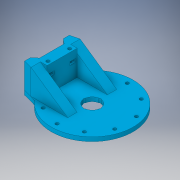
# Autodesk Inventor part: 000.302 - Кожух
Saved by Autodesk Inventor 2019 (Build 230136000, 136)
## iProperties
Created: 2020-03-19
Part Number: 000.302 - Кожух
Material: Пластик АБС
Document SubType Name: Modeling
Designer: user
Density: 1.06 g/cm^3
Appearance: Небесно-голубой — нейтральный
Author: user
Autodesk Inventor part; units mm, degrees
ref_plane "YZ Plane" through (0, 0, 0) normal (1, 0, 0) x (0, 1, 0)
ref_plane "XZ Plane" through (0, 0, 0) normal (0, 1, 0) x (-1, 0, 0)
sketch "Эскиз12" plane through (0, 0, 0) normal (0, 1, 0) x (-1, 0, 0)
  line L0 (114.5, 15) -> (114.5, 11.5)
  line L1 (114.5, 11.5) -> (114.5, -11.5)
  line L2 (114.5, -11.5) -> (114.5, -15)
  line L3 (114.5, -15) -> (108.5, -20.1)
  line L4 (108.5, -20.1) -> (55.4, -20.1)
  line L5 (55.4, -20.1) -> (49.4, -15)
  line L6 (49.4, -15) -> (49.4, 15)
  line L7 (49.4, 15) -> (55.4, 20.1)
  line L8 (55.4, 20.1) -> (108.5, 20.1)
  line L9 (108.5, 20.1) -> (114.5, 15)
  arc A0 (-1.6711, 9.8594) -> (-9.8594, 1.6711) centre (0, 0) ccw
  arc A1 (1.6711, 9.8594) -> (-1.6711, 9.8594) centre (0, 8) ccw
  arc A2 (9.8594, 1.6711) -> (1.6711, 9.8594) centre (0, 0) ccw
  arc A3 (9.8594, -1.6711) -> (9.8594, 1.6711) centre (8, 0) ccw
  arc A4 (1.6711, -9.8594) -> (9.8594, -1.6711) centre (0, 0) ccw
  arc A5 (-1.6711, -9.8594) -> (1.6711, -9.8594) centre (0, -8) ccw
  arc A6 (-9.8594, -1.6711) -> (-1.6711, -9.8594) centre (0, 0) ccw
  arc A7 (-9.8594, 1.6711) -> (-9.8594, -1.6711) centre (-8, 0) ccw
  circle A8 centre (0, 43) radius 2
  circle A9 centre (-25.2748, 34.7877) radius 2
  circle A10 centre (-40.8954, 13.2877) radius 2
  circle A11 centre (-40.8954, -13.2877) radius 2
  circle A12 centre (-25.2748, -34.7877) radius 2
  circle A13 centre (0, -43) radius 2
  circle A14 centre (25.2748, -34.7877) radius 2
  circle A15 centre (40.8954, -13.2877) radius 2
  circle A16 centre (40.8954, 13.2877) radius 2
  circle A17 centre (25.2748, 34.7877) radius 2
  arc A18 (38.3107, 32.1293) -> (38.3107, -32.1293) centre (0, 0) ccw
  arc A19 (97.8335, -24.9059) -> (38.3107, -32.1293) centre (85.2244, -169.8586) ccw
  arc A20 (97.8335, -24.9059) -> (97.8335, 24.9059) centre (100, 0) ccw
  arc A21 (38.3107, 32.1293) -> (97.8335, 24.9059) centre (85.2244, 169.8586) ccw
  circle A22 centre (52.2, 11) radius 1.025
  circle A23 centre (52.2, -11) radius 1.025
  circle A24 centre (60, -17.3) radius 1.025
  circle A25 centre (60, 17.3) radius 1.025
  line L10 (55, -11.5) -> (55, 11.5)
  arc A26 (58, 14.5) -> (55, 11.5) centre (58, 11.5) ccw
  line L11 (58, 14.5) -> (111.5, 14.5)
  arc A27 (55, -11.5) -> (58, -14.5) centre (58, -11.5) ccw
  line L12 (111.5, -14.5) -> (58, -14.5)
  arc A28 (111.5, -14.5) -> (114.5, -11.5) centre (111.5, -11.5) ccw
  arc A29 (114.5, 11.5) -> (111.5, 14.5) centre (111.5, 11.5) ccw
  line L13 (40.8954, 13.2877) -> (40.8954, -13.2877)
  line L14 (36.8954, 18.5) -> (44.8954, 18.5)
  line L15 (44.8954, 18.5) -> (44.8954, -18.5)
  line L16 (44.8954, -18.5) -> (36.8954, -18.5)
  line L17 (36.8954, -18.5) -> (36.8954, 18.5)
  line L18 (36.8954, 18.5) -> (44.8954, -18.5) construction
  line L19 (44.8954, 18.5) -> (36.8954, -18.5) construction
  line L20 (44.8954, -18.5) -> (44.8954, -30.0593)
  line L21 (55.4, -20.1) -> (55.4, -27.448)
  line L22 (55.4, 20.1) -> (55.4, 27.448)
  line L23 (44.8954, 18.5) -> (44.8954, 30.0593)
  point P0 (40.8954, 0)
  dimension "d45" = 8
  dimension "d46" = 37
  constraints: 48 end point, 36 point on circle, 30 centre point, 3 midpoint, 3 parallel, 2 point on line, 2 vertical, 1 horizontal, 1 perpendicular
  measures "d45" distance of L15.end L16.end
  measures "d46" distance of L14.end L15.end
extrude "Выдавливание9" add sketch "Эскиз12" along normal blind 5 contours L7 L6 L5 L21 A19 L20 L15 L23 A21 L22 | L23 L14 L17 L16 L20 A19 A18 A21 | L15 L16 L17 L14
sketch "Эскиз13" plane through (0, 5, 0) normal (0, 1, 0) x (1, 0, 0)
  line L0 (-114.5, -15) -> (-114.5, -11.5)
  line L1 (-114.5, -11.5) -> (-114.5, 11.5)
  line L2 (-114.5, 11.5) -> (-114.5, 15)
  line L3 (-114.5, 15) -> (-108.5, 20.1)
  line L4 (-108.5, 20.1) -> (-55.4, 20.1)
  line L5 (-55.4, 20.1) -> (-49.4, 15)
  line L6 (-49.4, 15) -> (-49.4, -15)
  line L7 (-49.4, -15) -> (-55.4, -20.1)
  line L8 (-55.4, -20.1) -> (-108.5, -20.1)
  line L9 (-108.5, -20.1) -> (-114.5, -15)
  arc A0 (1.6711, -9.8594) -> (9.8594, -1.6711) centre (0, 0) ccw
  arc A1 (-1.6711, -9.8594) -> (1.6711, -9.8594) centre (0, -8) ccw
  arc A2 (-9.8594, -1.6711) -> (-1.6711, -9.8594) centre (0, 0) ccw
  arc A3 (-9.8594, 1.6711) -> (-9.8594, -1.6711) centre (-8, 0) ccw
  arc A4 (-1.6711, 9.8594) -> (-9.8594, 1.6711) centre (0, 0) ccw
  arc A5 (1.6711, 9.8594) -> (-1.6711, 9.8594) centre (0, 8) ccw
  arc A6 (9.8594, 1.6711) -> (1.6711, 9.8594) centre (0, 0) ccw
  arc A7 (9.8594, -1.6711) -> (9.8594, 1.6711) centre (8, 0) ccw
  circle A8 centre (0, -43) radius 2
  circle A9 centre (25.2748, -34.7877) radius 2
  circle A10 centre (40.8954, -13.2877) radius 2
  circle A11 centre (40.8954, 13.2877) radius 2
  circle A12 centre (25.2748, 34.7877) radius 2
  circle A13 centre (0, 43) radius 2
  circle A14 centre (-25.2748, 34.7877) radius 2
  circle A15 centre (-40.8954, 13.2877) radius 2
  circle A16 centre (-40.8954, -13.2877) radius 2
  circle A17 centre (-25.2748, -34.7877) radius 2
  arc A18 (-38.3107, -32.1293) -> (-38.3107, 32.1293) centre (0, 0) ccw
  arc A19 (-97.8335, 24.9059) -> (-38.3107, 32.1293) centre (-85.2244, 169.8586) ccw
  arc A20 (-97.8335, 24.9059) -> (-97.8335, -24.9059) centre (-100, 0) ccw
  arc A21 (-38.3107, -32.1293) -> (-97.8335, -24.9059) centre (-85.2244, -169.8586) ccw
  circle A22 centre (-52.2, -11) radius 1.025
  circle A23 centre (-52.2, 11) radius 1.025
  circle A24 centre (-60, 17.3) radius 1.025
  circle A25 centre (-60, -17.3) radius 1.025
  line L10 (-55, 11.5) -> (-55, -11.5)
  arc A26 (-58, -14.5) -> (-55, -11.5) centre (-58, -11.5) ccw
  line L11 (-58, -14.5) -> (-111.5, -14.5)
  arc A27 (-55, 11.5) -> (-58, 14.5) centre (-58, 11.5) ccw
  line L12 (-111.5, 14.5) -> (-58, 14.5)
  arc A28 (-111.5, 14.5) -> (-114.5, 11.5) centre (-111.5, 11.5) ccw
  arc A29 (-114.5, -11.5) -> (-111.5, -14.5) centre (-111.5, -11.5) ccw
  line L13 (-40.8954, -13.2877) -> (-40.8954, 13.2877)
  line L14 (-36.8954, -18.5) -> (-44.8954, -18.5)
  line L15 (-44.8954, -18.5) -> (-44.8954, 18.5)
  line L16 (-44.8954, 18.5) -> (-36.8954, 18.5)
  line L17 (-36.8954, 18.5) -> (-36.8954, -18.5)
  line L18 (-36.8954, -18.5) -> (-44.8954, 18.5) construction
  line L19 (-44.8954, -18.5) -> (-36.8954, 18.5) construction
  line L20 (-44.8954, 18.5) -> (-44.8954, 30.0593)
  line L21 (-55.4, 20.1) -> (-55.4, 27.448)
  line L22 (-55.4, -20.1) -> (-55.4, -27.448)
  line L23 (-44.8954, -18.5) -> (-44.8954, -30.0593)
  point P0 (0, 0)
  point P1 (-40.8954, 0)
  dimension "d49" = 8
  dimension "d50" = 37
  constraints: 48 end point, 36 point on circle, 30 centre point, 3 midpoint, 3 parallel, 2 point on line, 1 perpendicular
  measures "d49" distance of L15.end L16.end
  measures "d50" distance of L14.end L15.end
extrude "Выдавливание10" add sketch "Эскиз13" along normal blind 31 contours L7 L6 L5 L21 A19 L20 L15 L23 A21 L22 | L15 L16 L17 L14
sketch "Эскиз14" plane through (-36.8954, 5, 18.5) normal (1, 0, 0) x (0, 0, -1)
  line L0 (3.2123, 0) -> (3.2123, 31) projected
  line L1 (7.2123, 0) -> (7.2123, 31) projected
  line L2 (29.7877, 0) -> (29.7877, 31) projected
  line L3 (33.7877, 0) -> (33.7877, 31) projected
  line L4 (3.2123, 19.2083) -> (7.2123, 19.2083)
  line L5 (1.5123, 17.2083) -> (8.9123, 17.2083)
  line L6 (8.9123, 17.2083) -> (8.9123, 21.2083)
  line L7 (8.9123, 21.2083) -> (1.5123, 21.2083)
  line L8 (1.5123, 21.2083) -> (1.5123, 17.2083)
  line L9 (1.5123, 17.2083) -> (8.9123, 21.2083) construction
  line L10 (8.9123, 17.2083) -> (1.5123, 21.2083) construction
  line L11 (29.7877, 19.2083) -> (33.7877, 19.2083)
  line L12 (28.0877, 17.2083) -> (35.4877, 17.2083)
  line L13 (35.4877, 17.2083) -> (35.4877, 21.2083)
  line L14 (35.4877, 21.2083) -> (28.0877, 21.2083)
  line L15 (28.0877, 21.2083) -> (28.0877, 17.2083)
  line L16 (28.0877, 17.2083) -> (35.4877, 21.2083) construction
  line L17 (35.4877, 17.2083) -> (28.0877, 21.2083) construction
  point P0 (5.2123, 19.2083)
  point P1 (31.7877, 19.2083)
  dimension "d53" = 7.4
  dimension "d54" = 4
  dimension "d55" = 7.4
  dimension "d56" = 4
  constraints: 28 end point, 6 midpoint, 4 parallel, 4 perpendicular, 4 point on line, 2 horizontal
  measures "d53" distance of L7.end L6.end
  measures "d54" distance of L6.end L5.end
  measures "d55" distance of L14.end L13.end
  measures "d56" distance of L13.end L12.end
extrude "Выдавливание11" cut sketch "Эскиз14" against normal blind 8
sketch "Эскиз16" plane through (0, 5, 0) normal (0, 1, 0) x (1, 0, 0)
  line L0 (0, -18.5) -> (-11.559, -18.5)
  line L1 (-11.559, -18.5) -> (-11.559, -30.059)
  line L2 (-11.559, -30.059) -> (0, -30.059)
  line L3 (0, -30.059) -> (0, -18.5)
  point P0 (0, 0)
  point P1 (-5.7795, -24.2795)
  dimension "d60" = 11.559
  dimension "d61" = 11.559
  constraints: 8 end point, 2 parallel, 1 horizontal, 1 perpendicular
  measures "d60" distance of L2.end L1.end
  measures "d61" distance of L1.end L0.end
loft "Лофт1" add profiles "Эскиз16" section 2 edges at (-44.8954, 20.5, 18.5) (-44.8954, 36, 24.2797) (-44.8954, 20.5, 30.0593) (-44.8954, 5, 24.2797)
ref_plane "РабПлоскость2" through (-36.8954, 36, 0) normal (0, 0, -1) x (-1, 0, 0)
mirror "Зеркальное отражение2" about plane through (-36.8954, 36, 0) normal (0, 0, -1) of "Лофт1"
sketch "Эскиз17" plane through (0, 36, 0) normal (0, 1, 0) x (1, 0, 0)
  circle A0 centre (-40.8954, -13.2877) radius 2 projected
  circle A1 centre (-40.8954, 13.2877) radius 2 projected
  line L0 (-36.8954, -18.5) -> (-36.8954, 18.5) projected
  line L1 (-36.8954, 18.5) -> (-44.8954, 18.5) projected
  line L2 (-44.8954, 18.5) -> (-44.8954, 30.0593) projected
  arc A2 (-55.4, 27.448) -> (-44.8954, 30.0593) centre (-85.2244, 169.8586) ccw projected
  line L3 (-55.4, 27.448) -> (-55.4, 20.1) projected
  line L4 (-55.4, 20.1) -> (-49.4, 15) projected
  line L5 (-49.4, 15) -> (-49.4, -15) projected
  line L6 (-49.4, -15) -> (-55.4, -20.1) projected
  line L7 (-55.4, -20.1) -> (-55.4, -27.448) projected
  arc A3 (-44.8954, -30.0593) -> (-55.4, -27.448) centre (-85.2244, -169.8586) ccw projected
  line L8 (-44.8954, -30.0593) -> (-44.8954, -18.5) projected
  line L9 (-44.8954, -18.5) -> (-36.8954, -18.5) projected
  point P0 (0, 0)
